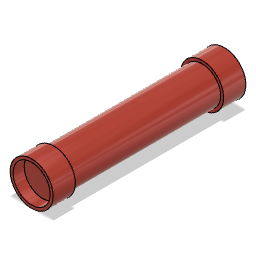
T-Stick (Autodesk Fusion 360 design; units mm, degrees)
Autodesk Fusion 360 part; units mm, degrees
sketch "Sketch1" plane through (0, 0, 0) normal (0, 0, 1) x (1, 0, 0)
  circle A0 centre (0, 0) radius 25
  circle A1 centre (0, 0) radius 29
  dimension "d3" = 50
  dimension "d4" = 4
  constraint coincident A0.centre A1.centre
  measures "d3" diameter of A0
extrude "Extrude1" add sketch "Sketch1" along normal blind 200 contours A0 makes body 1
extrude "Extrude2" add sketch "Sketch1" against normal blind 30 separate body makes body 2
extrude "Extrude3" add sketch "Sketch1" against normal blind 15 contours A0 bodies 1 2
sketch "Sketch2" plane through (0, 0, 200) normal (0, 0, 1) x (1, 0, 0)
  circle A0 centre (0, 0) radius 25
  circle A1 centre (0, 0) radius 29
  dimension "d9" = 4
extrude "Extrude4" add sketch "Sketch2" along normal blind 15 contours A0 bodies 1
extrude "Extrude5" add sketch "Sketch2" along normal blind 30 bodies 1
